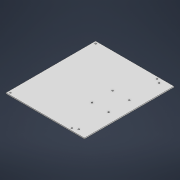
# Autodesk Inventor part: Obenplatte_vorne
Saved by Autodesk Inventor 2021 (Build 250183000, 183)
## iProperties
Created: 2021-02-01
Part Number: Obenplatte_vorne
Material: Generisch
Document SubType Name: Modeling
Designer: laure
Density: 1 g/cm^3
Appearance: Vorgabe
Author: laure
Autodesk Inventor part; units mm, degrees
ref_plane "YZ Plane" through (0, 0, 0) normal (1, 0, 0) x (0, 1, 0)
ref_plane "XZ Plane" through (0, 0, 0) normal (0, 1, 0) x (-1, 0, 0)
ref_plane "XY Plane" through (0, 0, 0) normal (0, 0, 1) x (1, 0, 0)
sketch "Skizze1" plane through (0, 0, 0) normal (0, 1, 0) x (-1, 0, 0)
  line L0 (87.5, -100) -> (-87.5, -100)
  line L1 (-87.5, -100) -> (-87.5, 100)
  line L2 (-87.5, 100) -> (87.5, 100)
  line L3 (87.5, 100) -> (87.5, -100)
  line L4 (0, -140) -> (0, 140) projected
  line L5 (122.5, 0) -> (-122.5, 0) projected
  point P0 (0, 0)
  dimension "d0" = 175
  dimension "d1" = 200
  constraints: 8 end point, 2 parallel, 1 horizontal, 1 perpendicular, 2 other
  measures "d0" distance of L1.end L2.end
  measures "d1" distance of L0.end L1.end
extrude "Extrusion1" add sketch "Skizze1" along normal blind 2
sketch "Skizze2" plane through (0, 2, 0) normal (0, 1, 0) x (1, 0, 0)
  circle A0 centre (54.5, 95) radius 1.6
  circle A1 centre (-82.5, 95) radius 1.6
  line L0 (0, 140) -> (0, -140) projected
  line L1 (122.5, 0) -> (-122.5, 0) projected
  line L2 (87.5, 100) -> (-87.5, 100) projected
  circle A2 centre (54.5, -95) radius 1.6
  circle A3 centre (-82.5, -95) radius 1.6
  line L3 (-87.5, 100) -> (-87.5, -100) projected
  line L4 (87.5, -100) -> (87.5, 100) projected
  point P0 (0, 0)
  dimension "d4" = 3.2
  dimension "d5" = 3.2
  dimension "d7" = 5
  dimension "d9" = 5
  dimension "d55" = 5
  dimension "d56" = 33
  constraints: 4 centre point, 2 symmetric about line, 2 other
  measures "d4" diameter of A0
  measures "d5" diameter of A1
  measures "d7" distance from line of L2 A0.centre
  measures "d9" distance from line of L2 A1.centre
  measures "d55" distance from line of L3 A1.centre
  measures "d56" distance from line of L4 A0.centre
extrude "Extrusion2" cut sketch "Skizze2" against normal up to surface (2 mm away) contours A0 | A1 | A2 | A3
sketch "Skizze3" plane through (0, 2, 0) normal (0, 1, 0) x (1, 0, 0)
  line L0 (0, 140) -> (0, -140) projected
  line L1 (122.5, 0) -> (-122.5, 0) projected
  line L2 (-87.5, -100) -> (87.5, -100) projected
  line L3 (-87.5, 100) -> (-87.5, -100) projected
  circle A0 centre (64.5, -89.5) radius 1.6
  line L4 (87.5, -100) -> (87.5, 100) projected
  circle A1 centre (64.5, -23) radius 1.6
  circle A2 centre (64.5, 23) radius 1.6
  line L5 (87.5, 100) -> (-87.5, 100) projected
  circle A3 centre (64.5, 89.5) radius 1.6
  circle A4 centre (27.5, -23) radius 1.6
  circle A5 centre (27.5, 23) radius 1.6
  point P0 (0, 0)
  dimension "d35" = 3.2
  dimension "d36" = 10.5
  dimension "d37" = 23
  dimension "d38" = 3.2
  dimension "d39" = 77
  dimension "d40" = 23
  dimension "d41" = 3.2
  dimension "d42" = 23
  dimension "d43" = 77
  dimension "d44" = 3.2
  dimension "d45" = 23
  dimension "d46" = 10.5
  dimension "d47" = 3.2
  dimension "d48" = 60
  dimension "d49" = 77
  dimension "d50" = 3.2
  dimension "d51" = 60
  dimension "d52" = 77
  constraints: 6 centre point
  measures "d35" diameter of A0
  measures "d36" distance from line of L2 A0.centre
  measures "d37" distance from line of L4 A0.centre
  measures "d38" diameter of A1
  measures "d39" distance from line of L2 A1.centre
  measures "d40" distance from line of L4 A1.centre
  measures "d41" diameter of A2
  measures "d42" distance from line of L4 A2.centre
  measures "d43" distance from line of L5 A2.centre
  measures "d44" diameter of A3
  measures "d45" distance from line of L4 A3.centre
  measures "d46" distance from line of L5 A3.centre
  measures "d47" diameter of A4
  measures "d48" distance from line of L4 A4.centre
  measures "d49" distance from line of L2 A4.centre
  measures "d50" diameter of A5
  measures "d51" distance from line of L4 A5.centre
  measures "d52" distance from line of L5 A5.centre
extrude "Extrusion3" cut sketch "Skizze3" against normal up to surface (2 mm away) contours A0 | A1 | A2 | A3 | A4 | A5
equation "\"d10\" = d6"
equation "\"d53\" = d48"
equation "\"d6\" = 42"
